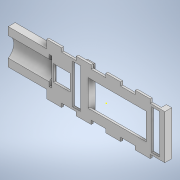
# Autodesk Inventor part: new base
Saved by Autodesk Inventor 2022 (Build 260153000, 153)
## iProperties
Created: 2022-04-14
Part Number: new base
Material: Generic
Document SubType Name: Modeling
Designer: vitalii
Density: 1 g/cm^3
Appearance: Default
Author: vitalii
Autodesk Inventor part; units mm, degrees
ref_plane "YZ Plane" through (0, 0, 0) normal (1, 0, 0) x (0, 1, 0)
ref_plane "XZ Plane" through (0, 0, 0) normal (0, 1, 0) x (-1, 0, 0)
ref_plane "XY Plane" through (0, 0, 0) normal (0, 0, 1) x (1, 0, 0)
sketch "Sketch1" plane through (0, 0, 0) normal (0, 0, 1) x (1, 0, 0)
  line L0 (-96.7048, 41.9035) -> (-96.7048, -42.0965)
  line L1 (-96.7048, -42.0965) -> (-72.3448, -42.0965)
  line L2 (-72.3448, -42.0965) -> (-72.3448, -36.0115)
  line L3 (-72.3448, -36.0115) -> (-48.7048, -36.0115)
  line L4 (-48.7048, -36.0115) -> (-48.7048, -42.0965)
  line L5 (-48.7048, -42.0965) -> (-24.3448, -42.0965)
  line L6 (-0.7048, -42.0965) -> (23.6552, -42.0965)
  line L7 (47.2952, -42.0965) -> (71.6552, -42.0965)
  line L8 (71.6552, -42.0965) -> (71.6552, -36.0115)
  line L9 (71.6552, -36.0115) -> (95.2952, -36.0115)
  line L10 (95.2952, -36.0115) -> (95.2952, 35.8185)
  line L11 (95.2952, 35.8185) -> (71.6552, 35.8185)
  line L12 (71.6552, 35.8185) -> (71.6552, 41.9035)
  line L13 (71.6552, 41.9035) -> (47.2952, 41.9035)
  line L14 (47.2952, 41.9035) -> (47.2952, 35.8185)
  line L15 (47.2952, 35.8185) -> (23.6552, 35.8185)
  line L16 (23.6552, 35.8185) -> (23.6552, 41.9035)
  line L17 (23.6552, 41.9035) -> (-0.7048, 41.9035)
  line L18 (-0.7048, 41.9035) -> (-0.7048, 35.8185)
  line L19 (-0.7048, 35.8185) -> (-24.3448, 35.8185)
  line L20 (-24.3448, 35.8185) -> (-24.3448, 41.9035)
  line L21 (-24.3448, 41.9035) -> (-48.7048, 41.9035)
  line L22 (-48.7048, 41.9035) -> (-48.7048, 35.8185)
  line L23 (-48.7048, 35.8185) -> (-72.3448, 35.8185)
  line L24 (-72.3448, 35.8185) -> (-72.3448, 41.9035)
  line L25 (-72.3448, 41.9035) -> (-96.7048, 41.9035)
  line L26 (-24.3448, -42.0965) -> (-24.3448, -36.0115)
  line L27 (-24.3448, -36.0115) -> (-0.7048, -36.0115)
  line L28 (-0.7048, -36.0115) -> (-0.7048, -42.0965)
  line L29 (23.6552, -42.0965) -> (23.6552, -36.0115)
  line L30 (23.6552, -36.0115) -> (47.2952, -36.0115)
  line L31 (47.2952, -36.0115) -> (47.2952, -42.0965)
  point P0 (0, 0)
  dimension "d0" = 84
  dimension "d1" = 24.36
  dimension "d2" = 23.64
  dimension "d3" = 24.36
  dimension "d5" = 24.36
  dimension "d8" = 23.64
  dimension "d9" = 71.83
  dimension "d10" = 23.64
  dimension "d11" = 6.085
  dimension "d12" = 6.085
  dimension "d13" = 6.085
  dimension "d14" = 24.36
  dimension "d15" = 23.64
  dimension "d16" = 24.36
  dimension "d17" = 23.64
  dimension "d18" = 24.36
  dimension "d19" = 23.64
  dimension "d20" = 24.36
  dimension "d21" = 23.64
  dimension "d22" = 23.64
  constraints: 64 end point, 20 perpendicular, 17 point on line, 3 vertical, 1 horizontal
  measures "d0" distance of L0.start L0.end
  measures "d1" distance of L0.end L1.end
  measures "d2" distance of L2.end L3.end
  measures "d3" distance of L4.end L5.end
  measures "d5" distance of L6.start L6.end
  measures "d8" distance of L26.end L27.end
  measures "d9" distance of L9.end L10.end
  measures "d10" distance of L8.end L9.end
  measures "d11" distance of L7.end L8.end
  measures "d12" distance of L27.end L6.start
  measures "d13" distance of L3.end L4.end
  measures "d14" distance of L24.end L0.start
  measures "d15" distance of L22.end L23.end
  measures "d16" distance of L20.end L21.end
  measures "d17" distance of L18.end L19.end
  measures "d18" distance of L16.end L17.end
  measures "d19" distance of L10.end L11.end
  measures "d20" distance of L12.end L13.end
  measures "d21" distance of L14.end L15.end
  measures "d22" distance of L29.end L30.end
extrude "Extrusion1" add sketch "Sketch1" against normal blind 3.25
sketch "Sketch2" plane through (0, 0, 0) normal (0, 0, 1) x (1, 0, 0)
  line L0 (-92.5348, 22.4285) -> (-92.5348, -22.6215)
  line L1 (-92.5348, -22.6215) -> (-88.4348, -22.6215)
  line L2 (-88.4348, -22.6215) -> (-88.4348, 22.4285)
  line L3 (-88.4348, 22.4285) -> (-92.5348, 22.4285)
  line L4 (-96.7048, 41.9035) -> (-96.7048, -42.0965) projected
  line L5 (-72.3448, 41.9035) -> (-96.7048, 41.9035) projected
  line L6 (-85.7648, 13.0835) -> (-85.7648, -13.2765)
  line L7 (-85.7648, -13.2765) -> (-58.5248, -13.2765)
  line L8 (-58.5248, -13.2765) -> (-58.5248, 13.0835)
  line L9 (-58.5248, 13.0835) -> (-85.7648, 13.0835)
  line L10 (-54.5548, 31.9735) -> (-54.5548, -32.1665)
  line L11 (-54.5548, -32.1665) -> (-41.9148, -32.1665)
  line L12 (-41.9148, -32.1665) -> (-41.9148, 31.9735)
  line L13 (-41.9148, 31.9735) -> (-54.5548, 31.9735)
  line L14 (-24.3448, 41.9035) -> (-48.7048, 41.9035) projected
  line L15 (-29.3448, 21.4335) -> (-29.3448, -21.6265)
  line L16 (-29.3448, -21.6265) -> (65.1152, -21.6265)
  line L17 (65.1152, -21.6265) -> (65.1152, 21.4335)
  line L18 (65.1152, 21.4335) -> (-29.3448, 21.4335)
  line L19 (73.8852, 31.9735) -> (73.8852, -32.1665)
  line L20 (73.8852, -32.1665) -> (86.5252, -32.1665)
  line L21 (86.5252, -32.1665) -> (86.5252, 31.9735)
  line L22 (71.6552, 35.8185) -> (95.2952, 35.8185) projected
  line L23 (86.5252, 31.9735) -> (73.8852, 31.9735)
  line L24 (95.2952, -36.0115) -> (95.2952, 35.8185) projected
  point P0 (0, 0)
  dimension "d25" = 4.17
  dimension "d26" = 4.1
  dimension "d27" = 45.05
  dimension "d28" = 19.475
  dimension "d29" = 10.94
  dimension "d30" = 26.36
  dimension "d31" = 27.24
  dimension "d32" = 42.15
  dimension "d33" = 28.82
  dimension "d34" = 64.14
  dimension "d35" = 12.64
  dimension "d36" = 9.93
  dimension "d37" = 67.36
  dimension "d38" = 43.06
  dimension "d39" = 94.46
  dimension "d40" = 20.47
  dimension "d41" = 64.14
  dimension "d42" = 12.64
  dimension "d43" = 3.845
  dimension "d44" = 8.77
  constraints: 40 end point, 15 perpendicular, 5 vertical
  measures "d25" distance between parallel lines of L4 L0
  measures "d26" distance of L2.end L0.start
  measures "d27" distance of L0.start L0.end
  measures "d28" distance between parallel lines of L3 L5
  measures "d29" distance between parallel lines of L4 L6
  measures "d30" distance of L6.start L6.end
  measures "d31" distance of L6.end L7.end
  measures "d32" distance between parallel lines of L4 L10
  measures "d33" distance between parallel lines of L5 L9
  measures "d34" distance of L10.start L10.end
  measures "d35" distance of L10.end L11.end
  measures "d36" distance between parallel lines of L14 L13
  measures "d37" distance between parallel lines of L4 L15
  measures "d38" distance of L15.start L15.end
  measures "d39" distance of L17.end L15.start
  measures "d40" distance between parallel lines of L14 L18
  measures "d41" distance of L20.end L21.end
  measures "d42" distance of L21.end L19.start
  measures "d43" distance between parallel lines of L22 L23
  measures "d44" distance between parallel lines of L24 L21
extrude "Extrusion2" cut sketch "Sketch2" against normal blind 4
sketch "Sketch3" plane through (0, 0, 0) normal (0, 0, 1) x (1, 0, 0)
  line L0 (-121.7905, 18.4035) -> (-90.4348, 18.4035)
  line L1 (-90.4348, 18.4035) -> (-90.4348, -18.5965)
  line L2 (-88.4348, 22.4285) -> (-88.4348, -22.6215) projected
  line L3 (-90.4348, -18.5965) -> (-121.7905, -18.5965)
  line L4 (-121.7905, -18.5965) -> (-121.7905, 18.4035)
  line L5 (-72.3448, 41.9035) -> (-96.7048, 41.9035) projected
  point P0 (0, 0)
  dimension "d47" = 37
  dimension "d48" = 23.5
  dimension "d49" = 2
  constraints: 8 end point, 2 perpendicular, 1 horizontal, 1 parallel
  measures "d47" distance of L3.end L0.start
  measures "d48" distance between parallel lines of L5 L0
  measures "d49" distance between parallel lines of L2 L1
extrude "Extrusion3" cut sketch "Sketch3" against normal blind 4
sketch "Sketch9" plane through (0, 0, 0) normal (0, 0, 1) x (1, 0, 0)
  line L0 (-92.5348, 28.4035) -> (-92.5348, -28.5965)
  line L1 (-92.5348, -28.5965) -> (-159.1348, -28.5965)
  line L2 (-159.1348, -28.5965) -> (-159.1348, 28.4035)
  line L3 (-159.1348, 28.4035) -> (-92.5348, 28.4035)
  line L4 (-92.5348, 18.4035) -> (-92.5348, 22.4285) projected
  line L5 (-72.3448, 41.9035) -> (-96.7048, 41.9035) projected
  line L6 (-96.7048, -42.0965) -> (-72.3448, -42.0965) projected
  point P0 (0, 0)
  dimension "d64" = 0
  dimension "d65" = 13.5
  dimension "d66" = 13.5
  dimension "d67" = 66.6
  constraints: 8 end point, 3 perpendicular, 1 vertical
  measures "d64" distance between parallel lines of L4 L0
  measures "d65" distance between parallel lines of L5 L3
  measures "d66" distance between parallel lines of L6 L1
  measures "d67" distance of L0.end L1.end
extrude "Extrusion6" add sketch "Sketch9" against normal blind 11.25
sketch "Sketch10" plane through (-159.1348, -28.5965, 0) normal (-1, 0, 0) x (0, 0, 1)
  circle A0 centre (9.5, 28.5) radius 18.5
  line L0 (0, 70.5) -> (-3.25, 70.5) projected
  line L1 (-11.25, 0) -> (-11.25, 57) projected
  point P0 (0, 28.5965)
  dimension "d70" = 42
  dimension "d71" = 37
  dimension "d72" = 20.75
  constraints: 1 centre point
  measures "d70" distance from line of L0 A0.centre
  measures "d71" diameter of A0
  measures "d72" distance from line of A0.centre L1
extrude "Extrusion7" cut sketch "Sketch10" against normal blind 66.6
sketch "Sketch11" plane through (0, 0, 0) normal (0, 0, 1) x (1, 0, 0)
  point P0 (0, 0)
sketch "Sketch12" plane through (0, 0, 0) normal (0, 0, 1) x (1, 0, 0)
  line L0 (86.5252, 35.8185) -> (86.5252, -36.0115)
  line L1 (86.5252, -36.0115) -> (95.2952, -36.0115)
  line L2 (95.2952, -36.0115) -> (95.2952, 35.8185)
  line L3 (95.2952, 35.8185) -> (86.5252, 35.8185)
  line L4 (95.2952, -36.0115) -> (95.2952, 35.8185) projected
  line L5 (95.2952, 35.8185) -> (71.6552, 35.8185) projected
  line L6 (86.5252, 31.9735) -> (86.5252, -32.1665) projected
  line L7 (71.6552, -36.0115) -> (95.2952, -36.0115) projected
  line L8 (-41.9148, 12.1175) -> (-41.9148, 35.8185)
  line L9 (-41.9148, 35.8185) -> (-41.9148, -36.0115)
  line L10 (-41.9148, -36.0115) -> (-29.3448, -36.0115)
  line L11 (-41.9148, 31.9735) -> (-41.9148, -32.1665) projected
  line L12 (-29.3448, -36.0115) -> (-29.3448, 35.8185)
  line L13 (-29.3448, -21.6265) -> (-29.3448, 21.4335) projected
  line L14 (-29.3448, 35.8185) -> (-41.9148, 35.8185)
  line L15 (-0.7048, 35.8185) -> (-24.3448, 35.8185) projected
  line L16 (-24.3448, -36.0115) -> (-0.7048, -36.0115) projected
  point P0 (0, 0)
  dimension "d75" = 0
  dimension "d76" = 0
  dimension "d77" = 0
  dimension "d78" = 0
  dimension "d79" = 0
  dimension "d80" = 0
  dimension "d81" = 0
  dimension "d82" = 0
  constraints: 18 end point, 5 perpendicular, 2 vertical, 1 collinear, 1 point on line
  measures "d75" distance between parallel lines of L5 L3
  measures "d76" distance between parallel lines of L6 L0
  measures "d77" distance between parallel lines of L4 L2
  measures "d78" distance between parallel lines of L7 L1
  measures "d79" distance between parallel lines of L15 L14
  measures "d80" distance between parallel lines of L16 L10
  measures "d81" distance between parallel lines of L11 L9
  measures "d82" distance between parallel lines of L13 L12
extrude "Extrusion8" add sketch "Sketch12" against normal blind 11.25
body "Solid1"
